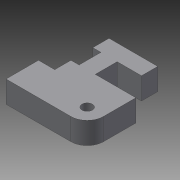
# Autodesk Inventor part: Carriage_Belt_Lock
Saved by Autodesk Inventor 2014 (Build 180170000, 170)
## iProperties
Created: 2014-08-27
Part Number: Carriage_Belt_Lock
Material: Generic
Document SubType Name: Modeling
Designer: ThatOtherGuy
Density: 1 g/cm^3
Appearance: Default
Author: ThatOtherGuy
Autodesk Inventor part; units mm, degrees
ref_plane "YZ Plane" through (0, 0, 0) normal (1, 0, 0) x (0, 1, 0)
ref_plane "XZ Plane" through (0, 0, 0) normal (0, 1, 0) x (-1, 0, 0)
ref_plane "XY Plane" through (0, 0, 0) normal (0, 0, 1) x (1, 0, 0)
sketch "Sketch1" plane through (0, 0, 0) normal (0, 0, 1) x (1, 0, 0)
  line L0 (25, 0) -> (0, 0)
  line L1 (0, 0) -> (0, 10)
  line L2 (0, 10) -> (5, 10)
  line L3 (25, 0) -> (25, 15)
  circle A0 centre (20, 5) radius 1.6
  line L4 (5, 10) -> (5, 15)
  line L5 (7.5, 15) -> (7.5, 21.731)
  line L6 (7.5, 21.731) -> (5, 21.731)
  line L7 (5, 21.731) -> (5, 26.731)
  line L8 (5, 26.731) -> (20, 26.731)
  line L9 (20, 26.731) -> (20, 21.731)
  line L10 (20, 21.731) -> (15, 21.731)
  line L11 (15, 21.731) -> (15, 15)
  line L12 (5, 15) -> (7.5, 15)
  line L13 (15, 15) -> (25, 15)
  dimension "d0" = 10
  dimension "d8" = 5
  dimension "d9" = 25
  dimension "d12" = 5
  dimension "d13" = 5
  dimension "d20" = 3.2
  dimension "d22" = 7.5
  dimension "d23" = 2.5
  dimension "d24" = 15
  dimension "d25" = 5
  dimension "d26" = 6.731
  dimension "d27" = 15
  constraints: 30 end point, 9 parallel, 6 perpendicular, 3 collinear, 1 centre point, 1 coincident, 1 vertical
  measures "d0" distance of L0.end L1.end
  measures "d8" distance of L1.end L2.end
  measures "d9" distance of L0.start L0.end
  measures "d12" distance from line of L3 A0.centre
  measures "d13" distance from line of L0 A0.centre
  measures "d20" diameter of A0
  measures "d22" distance between parallel lines of L5 L11
  measures "d23" distance between parallel lines of L4 L5
  measures "d24" distance of L7.end L8.end
  measures "d25" distance of L8.end L9.end
  measures "d26" distance of L10.end L11.end
  measures "d27" distance between parallel lines of L0 L13
extrude "Extrusion1" add sketch "Sketch1" along normal blind 6.731
fillet "Fillet1" radius 5 1 edges at (25, 0, 3.3655)
equation "\"d8\" = d3"
equation "\"d12\" = d13"
equation "\"d26\" = THICKB"
equation "\"d15\" = THICKB"
equation "\"THICKA\" = 3.175"
equation "\"THICKB\" = 6.731"
equation "\"THICKC\" = 12.7"
equation "\"MAGDIA\" = 9.5"
equation "\"BALLDIA\" = 12"
equation "\"d3\" = 5"
body "Solid1"
